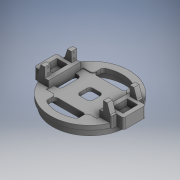
# Autodesk Inventor part: Swivel Top
Saved by Autodesk Inventor 2020.5 (Build 245400000, 400)
## iProperties
Created: 2023-04-01
Part Number: Swivel Top
Material: Generic
Document SubType Name: Modeling
Designer: Wes
Density: 1 g/cm^3
Appearance: Default
Author: Wes
Autodesk Inventor part; units mm, degrees
ref_plane "YZ Plane" through (0, 0, 0) normal (1, 0, 0) x (0, 1, 0)
ref_plane "XZ Plane" through (0, 0, 0) normal (0, 1, 0) x (-1, 0, 0)
ref_plane "XY Plane" through (0, 0, 0) normal (0, 0, 1) x (1, 0, 0)
sketch "Sketch1" plane through (0, 0, 0) normal (0, 0, 1) x (1, 0, 0)
  circle A0 centre (0, 0) radius 74
  dimension "d0" = 148
  constraints: 1 centre point, 1 coincident
  measures "d0" diameter of A0
extrude "Extrusion1" add sketch "Sketch1" along normal blind 8
sketch "Sketch2" plane through (0, 0, 8) normal (0, 0, 1) x (1, 0, 0)
  line L0 (0, 0) -> (0, -55) construction
  line L1 (0, 0) -> (0, 55) construction
  line L2 (0, -55) -> (0, -48) construction
  line L3 (0, -48) -> (-30, -48) construction
  line L4 (0, -48) -> (30, -48) construction
  line L5 (-30, -48) -> (30, -48)
  line L6 (30, -48) -> (30, -71)
  line L7 (30, -71) -> (-30, -71)
  line L8 (-30, -71) -> (-30, -48)
  line L9 (0, -71) -> (0, -84) construction
  line L10 (0, -84) -> (-21, -84) construction
  line L11 (0, -84) -> (21, -84) construction
  line L12 (-21, -84) -> (21, -84)
  line L13 (21, -84) -> (21, -71)
  line L14 (21, -71) -> (-21, -71)
  line L15 (-21, -71) -> (-21, -84)
  dimension "d3" = 55
  dimension "d5" = 7
  dimension "d7" = 30
  dimension "d8" = 60
  dimension "d9" = 23
  dimension "d10" = 13
  dimension "d11" = 21
  dimension "d13" = 42
  dimension "d14" = 13
  dimension "d15" = 60
  constraints: 32 end point, 6 horizontal, 4 parallel, 3 vertical, 2 perpendicular, 1 midpoint, 1 point on line
  measures "d3" distance of L0.start L0.end
  measures "d5" distance of L0.end L2.end
  measures "d7" distance of L2.end L4.end
  measures "d8" distance of L6.end L7.end
  measures "d9" distance of L5.end L6.end
  measures "d10" distance of L9.start L9.end
  measures "d11" distance of L9.end L10.end
  measures "d13" distance of L14.end L13.end
  measures "d14" distance of L13.end L12.end
  measures "d15" distance of L5.end L3.end
extrude "Extrusion2" add sketch "Sketch2" along normal blind 12 and the other way blind 8
sketch "Sketch3" plane through (0, 0, 20) normal (0, 0, 1) x (1, 0, 0)
  line L0 (30, -48) -> (-30, -48) construction
  line L1 (0, -48) -> (0, -55) construction
  line L2 (0, -55) -> (20.2, -55) construction
  line L3 (0, -55) -> (-20.2, -55) construction
  line L4 (20.2, -55) -> (30, -55)
  line L5 (30, -55) -> (30, -62.5)
  line L6 (30, -62.5) -> (20.2, -62.5)
  line L7 (20.2, -62.5) -> (20.2, -55)
  line L8 (-30, -48) -> (-30, -71) projected
  line L9 (-20.2, -55) -> (-30, -55)
  line L10 (-30, -55) -> (-30, -62.5)
  line L11 (-30, -62.5) -> (-20.2, -62.5)
  line L12 (-20.2, -62.5) -> (-20.2, -55)
  point P0 (0, 0)
  dimension "d20" = 7
  dimension "d21" = 20.2
  dimension "d23" = 40.4
  dimension "d24" = 9.8
  dimension "d25" = 7.5
  constraints: 22 end point, 4 horizontal, 4 parallel, 2 perpendicular, 1 midpoint, 1 point on line, 1 vertical
  measures "d20" distance of L1.start L1.end
  measures "d21" distance of L1.end L2.end
  measures "d23" distance of L2.end L3.end
  measures "d24" distance of L5.end L6.end
  measures "d25" distance of L4.end L5.end
extrude "Extrusion3" add sketch "Sketch3" along normal blind 18.5
sketch "Sketch4" plane through (-30, -55, 20) normal (0, 1, 0) x (1, 0, 0)
  line L0 (50.2, -18.5) -> (60, -18.5) construction
  line L1 (54.1927, -18.5) -> (54.1927, -14.845) construction
  line L2 (54.1927, -18.5) -> (57.8477, -18.5) construction
  line L3 (50.2, 0) -> (50.2, -18.5) construction
  line L4 (50.2, -14.845) -> (54.3, -14.845) construction
  line L5 (50.2, -14.845) -> (54.3, -14.845) construction
  circle A0 centre (54.3, -14.845) radius 1.275
  line L6 (54.3, -14.845) -> (54.3, -5.025) construction
  circle A1 centre (54.3, -5.025) radius 1.275
  line L7 (9, 0) -> (51, 0) construction
  line L8 (30, 0) -> (30, -30.1945) construction
  circle A2 centre (5.7, -14.845) radius 1.275
  circle A3 centre (5.7, -5.025) radius 1.275
  point P0 (30, 20)
  dimension "d28" = 3.655
  dimension "d30" = 4.1
  dimension "d32" = 2.55
  dimension "d33" = 9.82
  dimension "d34" = 2.55
  constraints: 12 end point, 4 centre point, 3 horizontal, 3 vertical, 2 coincident, 2 equal length, 2 point on line, 2 symmetric about line, 1 midpoint, 2 other
  measures "d28" distance of L1.start L1.end
  measures "d30" distance of L4.start L4.end
  measures "d32" diameter of A0
  measures "d33" distance of L6.start L6.end
  measures "d34" diameter of A1
extrude "Extrusion4" cut sketch "Sketch4" against normal blind 4.5
mirror "Mirror1" about plane through (0, 0, 0) normal (0, 1, 0) of "Extrusion2", "Extrusion3", "Extrusion4"
sketch "Sketch5" plane through (0, 0, 8) normal (0, 0, 1) x (1, 0, 0)
  line L0 (-30, 0) -> (-35, 0) construction
  line L1 (30, 0) -> (35, 0) construction
  line L2 (-35, -48) -> (35, -48)
  line L3 (35, -48) -> (35, 48)
  line L4 (35, 48) -> (-35, 48)
  line L5 (-35, 48) -> (-35, -48)
  point P0 (0, 0)
  dimension "d37" = 5
  dimension "d38" = 5
  constraints: 12 end point, 3 horizontal, 2 parallel, 1 perpendicular
  measures "d37" distance of L0.start L0.end
  measures "d38" distance of L1.start L1.end
extrude "Extrusion5" cut sketch "Sketch5" against normal blind 1.5
sketch "Sketch6" plane through (0, 0, 0) normal (0, 0, -1) x (-1, 0, 0)
  line L0 (-28.5, -28.5) -> (28.5, -28.5)
  line L1 (28.5, -28.5) -> (28.5, 28.5)
  line L2 (28.5, 28.5) -> (-28.5, 28.5)
  line L3 (-28.5, 28.5) -> (-28.5, -28.5)
  line L4 (-28.5, -28.5) -> (28.5, 28.5) construction
  line L5 (28.5, -28.5) -> (-28.5, 28.5) construction
  line L6 (-36.5, -36.5) -> (36.5, -36.5)
  line L7 (36.5, -36.5) -> (36.5, 36.5)
  line L8 (36.5, 36.5) -> (-36.5, 36.5)
  line L9 (-36.5, 36.5) -> (-36.5, -36.5)
  line L10 (-36.5, -36.5) -> (36.5, 36.5) construction
  line L11 (36.5, -36.5) -> (-36.5, 36.5) construction
  point P0 (0, 0)
  dimension "d41" = 57
  dimension "d42" = 57
  dimension "d43" = 73
  dimension "d44" = 73
  constraints: 24 end point, 4 midpoint, 4 parallel, 2 horizontal, 2 perpendicular
  measures "d41" distance of L2.end L1.end
  measures "d42" distance of L1.end L0.end
  measures "d43" distance of L8.end L7.end
  measures "d44" distance of L7.end L6.end
extrude "Extrusion6" add sketch "Sketch6" along normal blind 6
sketch "Sketch7" plane through (0, 0, 0) normal (0, 0, -1) x (-1, 0, 0)
  line L0 (-28.5, -28.5) -> (28.5, -28.5) construction
  line L1 (-16.506, -28.5) -> (-16.506, -20.5) construction
  line L2 (-16.506, -28.5) -> (-8.506, -28.5) construction
  line L3 (-28.5, 28.5) -> (-28.5, -28.5) construction
  line L4 (-28.5, -20.5) -> (-20.5, -20.5) construction
  line L5 (-28.5, -20.5) -> (-20.5, -20.5) construction
  circle A0 centre (-20.5, -20.5) radius 1.275
  circle A1 centre (20.5, -20.5) radius 1.275
  circle A2 centre (20.5, 20.5) radius 1.275
  circle A3 centre (-20.5, 20.5) radius 1.275
  point P0 (0, 0)
  dimension "d47" = 8
  dimension "d52" = 8
  dimension "d54" = 2.55
  dimension "d57" = 360
  constraints: 8 end point, 4 centre point, 3 horizontal, 2 equal length, 2 point on line, 1 coincident, 1 vertical, 9 other
  measures "d47" distance of L1.start L1.end
  measures "d52" distance of L4.start L4.end
  measures "d54" diameter of A0
extrude "Extrusion7" cut sketch "Sketch7" against normal blind 3.5
sketch "Sketch8" plane through (0, 0, 0) normal (0, 0, -1) x (-1, 0, 0)
  circle A0 centre (0, 0) radius 70
  circle A1 centre (0, 0) radius 66
  dimension "d61" = 140
  dimension "d62" = 132
  constraints: 2 centre point, 2 coincident
  measures "d61" diameter of A0
  measures "d62" diameter of A1
extrude "Extrusion8" add sketch "Sketch8" along normal blind 12
sketch "Sketch10" plane through (0, 0, 20) normal (0, 0, 1) x (1, 0, 0)
  line L0 (21, -84) -> (-21, -84) construction
  line L1 (0, -84) -> (0, -76) construction
  line L2 (35, -48) -> (-35, -48) construction
  line L3 (0, -48) -> (0, -56) construction
  line L4 (0, -48) -> (8, -48) construction
  line L5 (-21, -84) -> (-21, -71) construction
  line L6 (-21, -71) -> (-14, -71) construction
  line L7 (21, -71) -> (21, -84) construction
  line L8 (21, -71) -> (14, -71) construction
  line L9 (-35, -48) -> (-35, 48) construction
  line L10 (-35, 0) -> (35, 0) construction
  line L11 (35, 48) -> (35, -48) construction
  line L12 (-14, -76) -> (14, -76)
  line L13 (14, -76) -> (14, -56)
  line L14 (14, -56) -> (-14, -56)
  line L15 (-14, -56) -> (-14, -76)
  line L16 (-14, 76) -> (14, 76)
  line L17 (14, 76) -> (14, 56)
  line L18 (14, 56) -> (-14, 56)
  line L19 (-14, 56) -> (-14, 76)
  point P0 (0, 0)
  dimension "d84" = 10
  dimension "d70" = 8
  dimension "d71" = 8
  dimension "d73" = 7
  dimension "d74" = 7
  constraints: 28 end point, 4 horizontal, 4 midpoint, 4 symmetric about line, 2 parallel, 2 perpendicular, 2 vertical
  measures "d70" distance of L1.start L1.end
  measures "d71" distance of L3.start L3.end
  measures "d73" distance of L5.end L6.end
  measures "d74" distance of L7.start L8.end
extrude "Extrusion9" cut sketch "Sketch10" against normal blind 12
sketch "Sketch9" plane through (0, 0, 20) normal (0, 0, 1) x (1, 0, 0)
  circle A0 centre (0, 0) radius 66 construction
  circle A1 centre (0, 0) radius 70 construction
  line L0 (36.5, -36.5) -> (-36.5, -36.5) construction
  line L1 (-36.5, -36.5) -> (-36.5, 36.5) construction
  line L2 (-36.5, 36.5) -> (36.5, 36.5) construction
  line L3 (36.5, 36.5) -> (36.5, -36.5) construction
  line L4 (36.5, -36.5) -> (-36.5, 36.5) construction
  line L5 (-36.5, -36.5) -> (36.5, 36.5) construction
  circle A2 centre (0, 0) radius 74 construction
  line L6 (-28.5, -28.5) -> (28.5, -28.5) construction
  line L7 (28.5, -28.5) -> (28.5, 28.5) construction
  line L8 (28.5, 28.5) -> (-28.5, 28.5) construction
  line L9 (-28.5, 28.5) -> (-28.5, -28.5) construction
  line L10 (-28.5, -28.5) -> (28.5, 28.5) construction
  line L11 (28.5, -28.5) -> (-28.5, 28.5) construction
  circle A3 centre (-20.5, 20.5) radius 1.275 construction
  circle A4 centre (-20.5, -20.5) radius 1.275 construction
  circle A5 centre (20.5, -20.5) radius 1.275 construction
  circle A6 centre (20.5, 20.5) radius 1.275 construction
  circle A7 centre (0, 0) radius 66 construction
  line L12 (66, 0) -> (62, 0) construction
  line L13 (36.5, 36.5) -> (36.5, -36.5) construction
  line L14 (36.5, 0) -> (40.5, 0) construction
  line L15 (-12.5, -12.5) -> (12.5, -12.5)
  line L16 (12.5, -12.5) -> (12.5, 12.5)
  line L17 (12.5, 12.5) -> (-12.5, 12.5)
  line L18 (-12.5, 12.5) -> (-12.5, -12.5)
  line L19 (-12.5, -12.5) -> (12.5, 12.5) construction
  line L20 (12.5, -12.5) -> (-12.5, 12.5) construction
  line L21 (36.5, -36.5) -> (-36.5, -36.5) construction
  line L22 (0, -36.5) -> (0, -40.5) construction
  line L23 (30, -40.5) -> (20, -40.5) construction
  line L24 (-30, -40.5) -> (-20, -40.5) construction
  line L25 (35, -48) -> (-35, -48) projected
  line L26 (-20, -40.5) -> (20, -40.5)
  line L27 (20, -40.5) -> (20, -48)
  line L28 (20, -48) -> (-20, -48)
  line L29 (-20, -48) -> (-20, -40.5)
  line L30 (0, -106.0773) -> (0, 120.6178) construction
  line L31 (-88.4806, 0) -> (92.5805, 0) construction
  line L32 (40.5, -36.5) -> (40.5, -29.5) construction
  line L33 (40.5, 36.5) -> (40.5, 29.5) construction
  line L34 (40.5, -29.5) -> (40.5, 29.5)
  line L35 (40.5, -29.5) -> (54.5321, -29.5)
  line L36 (40.5, 29.5) -> (54.5321, 29.5)
  arc A8 (54.5321, -29.5) -> (54.5321, 29.5) centre (0, 0) ccw
  dimension "d65" = 132
  dimension "d66" = 140
  dimension "d67" = 73
  dimension "d68" = 73
  dimension "d69" = 148
  dimension "d77" = 57
  dimension "d78" = 57
  dimension "d79" = 4
  dimension "d80" = 4
  dimension "d81" = 25
  dimension "d82" = 25
  dimension "d83" = 4
  dimension "d84" = 10
  dimension "d85" = 10
  dimension "d86" = 7
  dimension "d87" = 7
  constraints: 68 end point, 10 horizontal, 9 parallel, 6 midpoint, 5 vertical, 4 centre point, 4 perpendicular, 3 coincident, 3 point on circle, 1 horizontal alignment, 1 point on line, 1 other
  measures "d65" diameter of A0
  measures "d66" diameter of A1
  measures "d67" distance of L1.end L2.end
  measures "d68" distance of L0.end L1.end
  measures "d69" diameter of A2
  measures "d77" distance of L8.end L7.end
  measures "d78" distance of L7.end L6.end
  measures "d79" distance of L12.start L12.end
  measures "d80" distance of L14.start L14.end
  measures "d81" distance of L17.end L16.end
  measures "d82" distance of L16.end L15.end
  measures "d83" distance of L22.start L22.end
  measures "d84" distance of L23.start L23.end
  measures "d85" distance of L24.start L24.end
  measures "d86" distance of L32.start L32.end
  measures "d87" distance of L33.start L33.end
sketch "Sketch12" plane through (0, 0, 8) normal (0, 0, 1) x (1, 0, 0)
  line L0 (-12.5, -12.5) -> (12.5, -12.5)
  line L1 (12.5, -12.5) -> (12.5, 12.5)
  line L2 (12.5, 12.5) -> (-12.5, 12.5)
  line L3 (-12.5, 12.5) -> (-12.5, -12.5)
  line L4 (-12.5, -12.5) -> (12.5, 12.5) construction
  line L5 (12.5, -12.5) -> (-12.5, 12.5) construction
  line L6 (30, -48) -> (-30, -48) construction
  line L7 (-30, -48) -> (-20, -48) construction
  line L8 (30, -55) -> (30, -48) construction
  line L9 (30, -48) -> (20, -48) construction
  circle A0 centre (0, 0) radius 66 construction
  line L10 (66, 0) -> (61, 0) construction
  line L11 (36.5, -36.5) -> (-36.5, -36.5) projected
  line L12 (-20, -48) -> (20, -48)
  line L13 (20, -48) -> (20, -36.5)
  line L14 (20, -36.5) -> (-20, -36.5)
  line L15 (-20, -36.5) -> (-20, -48)
  line L16 (36.5, 36.5) -> (-36.5, 36.5) projected
  line L17 (-35, 48) -> (35, 48) projected
  line L18 (-20, 36.5) -> (20, 36.5)
  line L19 (20, 36.5) -> (20, 48)
  line L20 (20, 48) -> (-20, 48)
  line L21 (-20, 48) -> (-20, 36.5)
  line L22 (36.5, 36.5) -> (36.5, -36.5) construction
  line L23 (36.5, -36.5) -> (36.5, -29.5) construction
  line L24 (36.5, -36.5) -> (43.5, -36.5) construction
  line L25 (36.5, 36.5) -> (36.5, 29.5) construction
  line L26 (36.5, -29.5) -> (36.5, 29.5)
  line L27 (36.5, -29.5) -> (53.3924, -29.5)
  line L28 (36.5, 29.5) -> (53.3924, 29.5)
  line L29 (-36.5, 36.5) -> (-36.5, -36.5) projected
  line L30 (-36.5, -29.5) -> (-36.5, 29.5)
  line L31 (-36.5, 29.5) -> (-53.3924, 29.5)
  line L32 (-36.5, -29.5) -> (-53.3924, -29.5)
  arc A1 (30, -53.1131) -> (53.3924, 29.5) centre (0, 0) ccw
  arc A2 (-53.3924, 29.5) -> (-53.3924, -29.5) centre (0, 0) ccw
  dimension "d100" = 25
  dimension "d101" = 25
  dimension "d102" = 10
  dimension "d103" = 10
  dimension "d104" = 5
  dimension "d105" = 7
  dimension "d107" = 7
  constraints: 52 end point, 9 point on line, 7 perpendicular, 6 horizontal, 6 parallel, 6 point on circle, 2 centre point, 2 midpoint, 1 coincident, 1 collinear, 1 horizontal alignment, 1 vertical, 1 other
  measures "d100" distance of L2.end L1.end
  measures "d101" distance of L1.end L0.end
  measures "d102" distance of L6.end L7.end
  measures "d103" distance of L6.start L9.end
  measures "d104" distance of L10.start L10.end
  measures "d105" distance of L11.start L23.end
  measures "d107" distance of L16.start L25.end
extrude "Extrusion11" cut sketch "Sketch12" against normal up to surface (8 mm away)
sketch "Sketch13" plane through (0, 0, 8) normal (0, 0, 1) x (1, 0, 0)
  line L0 (-36.5, 29.5) -> (-36.5, -29.5) projected
  line L1 (-35, -48) -> (-35, 48) projected
  line L2 (-36.5, -29.5) -> (-53.3924, -29.5) projected
  line L3 (-35, 29.5) -> (-36.5, 29.5)
  line L4 (-36.5, 29.5) -> (-36.5, -29.5)
  line L5 (-36.5, -29.5) -> (-35, -29.5)
  line L6 (-35, -29.5) -> (-35, 29.5)
  line L7 (35, 48) -> (35, -48) projected
  line L8 (36.5, -29.5) -> (36.5, 29.5) projected
  line L9 (35, -29.5) -> (36.5, -29.5)
  line L10 (36.5, -29.5) -> (36.5, 29.5)
  line L11 (36.5, 29.5) -> (35, 29.5)
  line L12 (35, 29.5) -> (35, -29.5)
  point P0 (0, 0)
  constraints: 16 end point, 4 parallel, 2 horizontal, 2 perpendicular, 2 point on line
extrude "Extrusion12" cut sketch "Sketch13" against normal up to surface (1.5 mm away)
draft "FaceDraft1" angle 18 pull direction (0, 0, 1) faces at (-26.7333, -62.5, 26.1667) (23.4667, -62.5, 26.1667) (-26.7333, 62.5, 26.1667) (23.4667, 62.5, 26.1667) fixed edges at (-25.1, -62.5, 38.5) (25.1, -62.5, 38.5) (-25.1, 62.5, 38.5) (25.1, 62.5, 38.5)
fillet "Fillet1" radius 4 8 edges at (21, -84, 10) (-21, -84, 10) (21, 84, 10) (-21, 84, 10) (30, 71, 10) (-30, 71, 10) (30, -71, 10) (-30, -71, 10)
fillet "Fillet2" radius 2 4 edges at (-24.9518, -68.511, 20) (24.9518, -68.511, 20) (24.9518, 68.511, 20) (-24.9518, 68.511, 20)
fillet "Fillet3" radius 6 20 edges at (-12.5, -12.5, 3.25) (-12.5, 12.5, 3.25) (12.5, 12.5, 3.25) (12.5, -12.5, 3.25) (-20, -36.5, 3.25) (20, -36.5, 3.25) (36.5, -29.5, 3.25) (36.5, 29.5, 3.25) (-20, 36.5, 3.25) (20, 36.5, 3.25) (-36.5, 29.5, 3.25) (-36.5, -29.5, 3.25) (53.3924, 29.5, 4) (53.3924, -29.5, 4) (-53.3924, 29.5, 4) (-53.3924, -29.5, 4) (35, 29.5, 7.25) (-35, 29.5, 7.25) (-35, -29.5, 7.25) (35, -29.5, 7.25)
body "Solid1"
